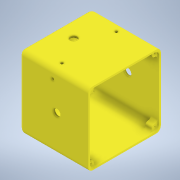
# Autodesk Inventor part: base_nasa
Saved by Autodesk Inventor 2021 (Build 250183000, 183)
## iProperties
Created: 2024-10-05
Part Number: base_nasa
Material: Generic
Document SubType Name: Modeling
Designer: hojan
Density: 1 g/cm^3
Appearance: Default
Author: hojan
Autodesk Inventor part; units mm, degrees
ref_plane "YZ Plane" through (0, 0, 0) normal (1, 0, 0) x (0, 1, 0)
sketch "Boceto1" plane through (0, 0, 0) normal (1, 0, 0) x (0, 1, 0)
  line L0 (-40, 40) -> (40, 40)
  line L1 (40, 40) -> (40, -40)
  line L2 (40, -40) -> (-40, -40)
  line L3 (-40, -40) -> (-40, 40)
  line L4 (-40, 40) -> (40, -40) construction
  line L5 (40, 40) -> (-40, -40) construction
  line L6 (-38, -38) -> (38, -38)
  line L7 (38, -38) -> (38, 38)
  line L8 (38, 38) -> (-38, 38)
  line L9 (-38, 38) -> (-38, -38)
  point P0 (0, 0)
  dimension "d2" = 80
  dimension "d3" = 80
  dimension "d4" = 2
  constraints: 20 end point, 4 parallel, 2 midpoint, 2 perpendicular, 1 horizontal, 3 other
  measures "d2" distance of L1.end L2.end
  measures "d3" distance of L0.end L1.end
  measures "d4" distance between parallel lines of L2 L6
extrude "Extrusión1" add sketch "Boceto1" along normal blind 76
sketch "Boceto2" plane through (0, 0, 0) normal (-1, 0, 0) x (0, 0, 1)
  line L0 (38, -38) -> (38, 38) projected
  line L1 (-38, -38) -> (38, -38)
  line L2 (38, -38) -> (38, 38)
  line L3 (38, 38) -> (-38, 38)
  line L4 (-38, 38) -> (-38, -38)
  line L5 (-38, -38) -> (38, 38) construction
  line L6 (38, -38) -> (-38, 38) construction
  point P0 (0, 0)
  constraints: 12 end point, 2 midpoint, 2 parallel, 1 horizontal, 1 perpendicular
extrude "Extrusión2" add sketch "Boceto2" against normal blind 2
fillet "Empalme1" radius 5 16 edges at (38, 40, 40) (38, -40, 40) (38, -40, -40) (38, 40, -40) (0, -40, 0) (0, 0, 40) (0, 40, 0) (0, 0, -40) (39, -38, -38) (2, 0, -38) (39, 38, -38) (39, 38, 38) (39, -38, 38) (2, 38, 0) (2, -38, 0) (2, 0, 38)
sketch "Boceto4" plane through (2, 0, 0) normal (1, 0, 0) x (0, 0, -1)
  line L0 (-38, 38) -> (38, 38) projected
  line L1 (-38, 38) -> (-18, 38)
  line L2 (-18, 38) -> (-18, 18)
  line L3 (-18, 18) -> (-38, 18)
  line L4 (-38, -38) -> (-38, 38) projected
  line L5 (-38, 38) -> (-36, 38)
  line L6 (-36, 38) -> (-36, 36)
  circle A0 centre (-36, 36) radius 1
  circle A1 centre (-32, 36) radius 1
  circle A2 centre (-28, 36) radius 1
  circle A3 centre (-24, 36) radius 1
  circle A4 centre (-20, 36) radius 1
  circle A5 centre (-36, 32) radius 1
  circle A6 centre (-32, 32) radius 1
  circle A7 centre (-28, 32) radius 1
  circle A8 centre (-24, 32) radius 1
  circle A9 centre (-20, 32) radius 1
  circle A10 centre (-36, 28) radius 1
  circle A11 centre (-32, 28) radius 1
  circle A12 centre (-28, 28) radius 1
  circle A13 centre (-24, 28) radius 1
  circle A14 centre (-20, 28) radius 1
  circle A15 centre (-36, 24) radius 1
  circle A16 centre (-32, 24) radius 1
  circle A17 centre (-28, 24) radius 1
  circle A18 centre (-24, 24) radius 1
  circle A19 centre (-20, 24) radius 1
  circle A20 centre (-36, 20) radius 1
  circle A21 centre (-32, 20) radius 1
  circle A22 centre (-28, 20) radius 1
  circle A23 centre (-24, 20) radius 1
  circle A24 centre (-20, 20) radius 1
  point P0 (0, 0)
  dimension "d45" = 20
  dimension "d46" = 20
  dimension "d47" = 2
  dimension "d48" = 2
  dimension "d49" = 2
  dimension "d52" = 4
  dimension "d59" = 4
  constraints: 25 centre point, 10 end point, 3 perpendicular, 3 point on line, 1 coincident, 1 horizontal, 1 vertical, 48 other
  measures "d45" distance of L0.start L1.end
  measures "d46" distance of L1.end L2.end
  measures "d47" distance of L0.start L5.end
  measures "d48" distance of L5.end L6.end
  measures "d49" diameter of A0
  measures "d52" distance of A0.centre A1.centre
  measures "d59" distance of A0.centre A5.centre
extrude "Extrusión4" cut sketch "Boceto4" against normal mid plane 8 contours A0 | A1 | A2 | A3 | A4 | A5 | A6 | A7 | A8 | A9 | A10 | A11 | A12 | A13 | A14 | A15 | A16 | A17 | A18 | A19 | A20 | A21 | A22 | A23 | A24
mirror "Simetría5" about plane through (0, 0, 0) normal (0, 0, 1) of "Extrusión4"
mirror "Simetría6" about plane through (0, 0, 0) normal (0, 1, 0) of "Extrusión4", "Simetría5"
ref_plane "Plano de trabajo3" through (74, 0, 0) normal (1, 0, 0) x (0, 0, -1)
sketch "Boceto5" plane through (74, 0, 0) normal (1, 0, 0) x (0, 0, -1)
  line L0 (-38, 38) -> (38, 38) projected
  line L1 (38, 38) -> (38, 35)
  line L2 (38, 38) -> (38, -38) projected
  line L3 (38, 35) -> (35, 35)
  circle A0 centre (35, 35) radius 1
  circle A1 centre (35, 35) radius 3
  line L4 (38, 38) -> (35, 38)
  point P0 (0, 0)
  dimension "d67" = 3
  dimension "d68" = 3
  dimension "d69" = 2
  constraints: 6 end point, 2 centre point, 2 coincident, 2 point on circle, 2 point on line, 1 perpendicular
  measures "d67" distance of L0.end L1.end
  measures "d68" distance of L1.end L3.end
  measures "d69" diameter of A0
extrude "Extrusión5" add sketch "Boceto5" against normal blind 7
fillet "Empalme2" radius 3 2 edges at (70.5, 34.1292, -37.8708) (70.5, 37.8708, -34.1292)
mirror "Simetría7" about plane through (0, 0, 0) normal (0, 1, 0) of "Extrusión5", "Empalme2"
mirror "Simetría8" about plane through (0, 0, 0) normal (0, 0, 1) of "Extrusión5", "Empalme2"
ref_plane "Plano de trabajo7" through (2, -33, -33) normal (0, 0.7071068, -0.7071068) x (0, 0.7071068, 0.7071068)
mirror "Simetría10" about plane through (2, -33, -33) normal (0, 0.7071068, -0.7071068) of "Extrusión5"
fillet "Empalme3" radius 3 2 edges at (70.5, -34.1292, 37.8708) (70.5, -37.8708, 34.1292)
sketch "Boceto6" plane through (5, 35, 40) normal (0, 0, 1) x (1, 0, 0)
  line L0 (62, 3) -> (2, 3) projected
  line L1 (32, 3) -> (32, -5)
  line L2 (62, -2) -> (2, -2) projected
  line L3 (32, 3) -> (40, 3) construction
  circle A0 centre (32, -5) radius 1.5
  point P0 (-5, -35)
  dimension "d74" = 8
  dimension "d75" = 90
  dimension "d76" = 3
  constraints: 4 end point, 2 perpendicular, 1 centre point, 1 coincident, 1 horizontal, 1 midpoint
  measures "d74" distance of L1.start L1.end
  measures "d75" angle of L1 L3
  measures "d76" diameter of A0
extrude "Extrusión6" cut sketch "Boceto6" against normal blind 100
sketch "Boceto7" plane through (5, 40, 35) normal (0, 1, 0) x (1, 0, 0)
  line L0 (33.5, 73) -> (30.5, 73) projected
  line L1 (32, 73) -> (32, 65)
  line L2 (32, 73) -> (40, 73) construction
  line L3 (2, -3) -> (62, -3) projected
  line L4 (32, -3) -> (32, 5)
  circle A0 centre (32, 5) radius 1.5
  circle A1 centre (32, 65) radius 1.5
  point P0 (-5, 35)
  dimension "d81" = 8
  dimension "d82" = 270
  dimension "d83" = 8
  dimension "d84" = 3
  dimension "d85" = 3
  constraints: 6 end point, 2 centre point, 2 coincident, 2 midpoint, 2 vertical, 1 horizontal, 1 perpendicular
  measures "d81" distance of L1.start L1.end
  measures "d83" distance of L4.start L4.end
  measures "d84" diameter of A0
  measures "d85" diameter of A1
extrude "Extrusión7" cut sketch "Boceto7" against normal blind 10
sketch "Boceto9" plane through (0, 0, 0) normal (-1, 0, 0) x (0, 0, 1)
  circle A0 centre (0, 0) radius 4
  dimension "d88" = 8
  constraints: 1 centre point, 1 coincident
  measures "d88" diameter of A0
extrude "Extrusión8" cut sketch "Boceto9" against normal blind 10
sketch "Boceto10" plane through (5, 40, 35) normal (0, 1, 0) x (1, 0, 0)
  line L0 (0, 70) -> (0, 0) projected
  line L1 (0, 35) -> (15, 35)
  circle A0 centre (15, 35) radius 4
  point P0 (-5, 35)
  dimension "d91" = 15
  dimension "d92" = 8
  constraints: 2 end point, 1 centre point, 1 coincident, 1 horizontal, 1 midpoint
  measures "d91" distance of L1.start L1.end
  measures "d92" diameter of A0
extrude "Extrusión9" cut sketch "Boceto10" against normal blind 100
sketch "Boceto12" plane through (5, 35, 40) normal (0, 0, 1) x (1, 0, 0)
  circle A0 centre (36.5, -35) radius 4
  point P0 (-5, -35)
  dimension "d95" = 8
  constraints: 1 centre point
  measures "d95" diameter of A0
extrude "Extrusión10" cut sketch "Boceto12" against normal blind 100
sketch "Boceto13" plane through (2, 32, 20) normal (1, 0, 0) x (0, 0, -1)
  line L0 (-13, -70) -> (53, -70) projected
  line L1 (20, -70) -> (20, -54)
  line L2 (18, -56) -> (22, -56)
  line L3 (22, -56) -> (22, -52)
  line L4 (22, -52) -> (18, -52)
  line L5 (18, -52) -> (18, -56)
  line L6 (18, -56) -> (22, -52) construction
  line L7 (22, -56) -> (18, -52) construction
  point P0 (20, -32)
  dimension "d98" = 16
  dimension "d100" = 4
  dimension "d101" = 4
  constraints: 14 end point, 3 midpoint, 2 parallel, 1 horizontal, 1 perpendicular, 1 vertical
  measures "d98" distance of L1.start L1.end
  measures "d100" distance of L4.end L3.end
  measures "d101" distance of L3.end L2.end
extrude "Extrusión11" cut sketch "Boceto13" against normal blind 100
